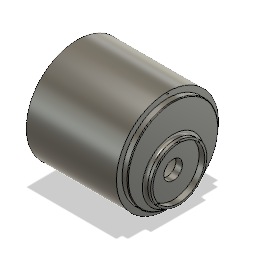
QWEwwe (5) (Autodesk Fusion 360 design; units mm, degrees)
Autodesk Fusion 360 part; units mm, degrees
sketch "Sketch1" plane through (0, 0, 0) normal (0, 0, 1) x (1, 0, 0)
sketch "Sketch2" plane through (0, 0, 0) normal (0, 0, 1) x (1, 0, 0)
  line L0 (0, 0) -> (-4.064, 0)
  line L1 (-403.86, 200.025) -> (-367.284, 200.025)
  line L2 (-91.44, 219.075) -> (-308.5474, 219.075)
  line L3 (-403.86, 200.025) -> (-403.86, 228.346)
  line L4 (-403.86, 228.346) -> (-4.064, 228.346)
  line L5 (-4.064, 131.699) -> (-4.064, 0)
  arc A0 (-4.064, 131.699) -> (-91.44, 219.075) centre (-91.44, 131.699) ccw
  line L6 (-403.86, 228.346) -> (0, 228.346)
  line L7 (0, 228.346) -> (0, 219.075)
  line L8 (0, 219.075) -> (0, 0)
  arc A1 (-308.5474, 219.075) -> (-367.284, 200.025) centre (-318.7192, 150.3616) ccw
  dimension "d10" = 87.376
  dimension "d11" = 403.86
  dimension "d12" = 9.271
  measures "d10" radius of A0
  measures "d11" distance of L0.start
revolve "Revolve1" add sketch "Sketch2" angle 360 about axis through (1.75, 0, 0) along (1, 0, 0)
sketch "Sketch3" plane through (0, 0, 0) normal (1, 0, 0) x (0, 0, -1)
  circle A0 centre (0, 0) radius 228.346
  line L0 (0, 228.346) -> (0, 203.073)
  circle A1 centre (0, 0) radius 203.073
  dimension "d16" = 25.273
extrude "Extrude1" add sketch "Sketch3" along normal blind 24.892 contours A1
sketch "Sketch4" plane through (24.892, 0, 0) normal (1, 0, 0) x (0, 0, -1)
  circle A0 centre (0, 0) radius 203.073
  circle A1 centre (0, -61.341) radius 125.476
  circle A2 centre (0, -61.341) radius 115.8875
  dimension "d20" = 231.775
  measures "d20" diameter of A2
chamfer "Chamfer1" distance 3.048 angle 45 1 edges at (24.892, -73.4343, 189.3305)
extrude "Extrude2" add sketch "Sketch4" along normal blind 25.4 contours A1
fillet "Fillet1" radius 11.938 1 edges at (24.892, -15.9669, 116.9847)
sketch "Sketch5" plane through (24.892, 0, 0) normal (1, 0, 0) x (0, 0, -1)
  circle A0 centre (0, -61.341) radius 115.8875
  circle A1 centre (0, -61.341) radius 41.5925
  dimension "d25" = 83.185
  measures "d25" diameter of A1
extrude "Extrude3" cut sketch "Sketch5" against normal blind 889 contours A1
sketch "Sketch6" plane through (-403.86, 0, 0) normal (-1, 0, 0) x (0, 0, 1)
  circle A0 centre (0, 0) radius 200.025
  circle A1 centre (0, 0) radius 228.346
  line L0 (0, 228.346) -> (0, 220.726)
  circle A2 centre (0, 220.726) radius 3.2004
  dimension "d28" = 7.62
  dimension "d29" = 6.4008
  measures "d29" diameter of A2
extrude "Extrude4" cut sketch "Sketch6" against normal blind 8.128 contours A2
sketch "Sketch7" plane through (0, 0, 0) normal (1, 0, 0) x (0, 0, -1)
  circle A0 centre (0, 0) radius 203.073
  circle A1 centre (0, 0) radius 228.346
  line L0 (0, 228.346) -> (0, 220.218)
  circle A2 centre (0, 220.218) radius 3.2004
  dimension "d32" = 8.128
  dimension "d33" = 6.4008
  measures "d33" diameter of A2
extrude "Extrude5" cut sketch "Sketch7" against normal blind 8.128 contours A2
sketch "Sketch8" plane through (50.292, 0, 0) normal (1, 0, 0) x (0, 0, -1)
  circle A0 centre (0, -61.341) radius 115.8875
  circle A1 centre (0, -61.341) radius 125.476
  circle A2 centre (0.0718, 59.2759) radius 4.7625
  dimension "d36" = 9.525
  measures "d36" diameter of A2
hole "Hole1" at (50.292, 59.2759, -0.0718) direction (-1, 0, 0) diameter 9.144 depth 25.4 tip angle 180
hole "Hole2" at (50.292, 16.31, -92.4949) direction (-1, 0, 0) diameter 9.144 depth 25.4 tip angle 180
hole "Hole3" at (50.292, 23.8114, 85.7159) direction (-1, 0, 0) diameter 9.144 depth 25.4 tip angle 180
hole "Hole4" at (50.292, -135.0672, 95.7736) direction (-1, 0, 0) diameter 9.144 depth 25.4 tip angle 180
hole "Hole5" at (50.292, -124.6176, -102.8884) direction (-1, 0, 0) diameter 9.144 depth 25.4 tip angle 180
equation "d12 = ( ( 17.98 - 17.25 ) / 2 ) * 1 in"
equation "d16 = ( 1.99 / 2 ) * 1 in"
